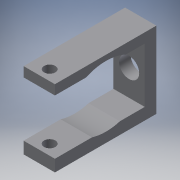
# Autodesk Inventor part: amt_dragster
Saved by Autodesk Inventor 2019 (Build 230136000, 136)
## iProperties
Created: 2024-05-02
Part Number: amt_dragster
Material: Generisch
Document SubType Name: Modeling
Designer: nic
Density: 1 g/cm^3
Appearance: Vorgabe
Author: nic
Autodesk Inventor part; units mm, degrees
ref_plane "YZ Plane" through (0, 0, 0) normal (1, 0, 0) x (0, 1, 0)
ref_plane "XZ Plane" through (0, 0, 0) normal (0, 1, 0) x (-1, 0, 0)
ref_plane "XY Plane" through (0, 0, 0) normal (0, 0, 1) x (1, 0, 0)
sketch "Skizze1" plane through (0, 0, 0) normal (0, 0, 1) x (1, 0, 0)
  line L0 (16.6415, 9.8457) -> (8.5751, 9.8457)
  line L1 (8.5751, 9.8457) -> (8.5751, -9.8457)
  line L2 (8.5751, -9.8457) -> (16.6415, -9.8457)
  line L3 (16.6415, -9.8457) -> (16.6415, 9.8457)
  line L4 (16.6415, 9.8457) -> (8.5751, -9.8457) construction
  line L5 (8.5751, 9.8457) -> (16.6415, -9.8457) construction
  circle A0 centre (12.6083, 0) radius 2.6
  point P0 (0, 0)
  dimension "d0" = 5.2
  constraints: 12 end point, 2 midpoint, 2 parallel, 1 centre point, 1 coincident, 1 horizontal, 1 perpendicular
  measures "d0" diameter of A0
extrude "Extrusion1" add sketch "Skizze1" along normal blind 3
sketch "Skizze2" plane through (0, 0, 3) normal (0, 0, 1) x (1, 0, 0)
  circle A0 centre (12.6083, 0) radius 2.6 construction
  line L0 (16.6415, 9.8457) -> (8.5751, 9.8457) construction
  line L1 (8.5751, 9.8457) -> (8.5751, -9.8457) construction
  line L2 (8.5751, -9.8457) -> (16.6415, -9.8457) construction
  line L3 (16.6415, -9.8457) -> (16.6415, 9.8457) construction
  line L4 (8.5751, 9.8457) -> (8.5751, -9.8457) projected
  line L5 (16.6415, -9.8457) -> (8.5751, -9.8457)
  line L6 (8.5751, -9.8457) -> (8.5751, -6.7929)
  line L7 (8.5751, -6.7929) -> (16.6415, -6.7929)
  line L8 (16.6415, -6.7929) -> (16.6415, -9.8457)
  line L9 (16.6415, -9.8457) -> (16.6415, 9.8457) projected
  line L10 (8.5751, 9.8457) -> (16.6415, 9.8457)
  line L11 (16.6415, 9.8457) -> (16.6415, 7.3365)
  line L12 (16.6415, 7.3365) -> (8.5751, 7.3365)
  line L13 (8.5751, 7.3365) -> (8.5751, 9.8457)
  point P0 (0, 0)
  constraints: 16 end point, 4 parallel, 2 horizontal, 2 perpendicular, 2 point on line
extrude "Extrusion2" add sketch "Skizze2" along normal blind 25 contours L10 L9 L12 L4 | L7 L8 L5 L4
sketch "Skizze3" plane through (8.5751, 7.3365, 3) normal (0, -1, 0) x (1, 0, 0)
  line L0 (8.0665, 0) -> (0, 0) projected
  line L1 (8.0665, 0) -> (8.0665, 25) projected
  line L2 (0, 25) -> (8.0665, 25) projected
  line L3 (0, 0) -> (0, 25) projected
  circle A0 centre (4.0332, 20.469) radius 1.4552
  point P0 (-8.5751, -3)
  constraints: 1 centre point
extrude "Extrusion3" cut sketch "Skizze3" along normal through all both and the other way through all contours A0
sketch "Skizze4" plane through (8.5751, -9.8457, 0) normal (0, -1, 0) x (1, 0, 0)
  line L0 (8.0665, 3) -> (8.0665, 28) projected
  line L1 (0, 3) -> (0, 28) projected
  line L2 (8.0665, 28) -> (0, 28)
  line L3 (0, 28) -> (0, 26.1511)
  line L4 (0, 26.1511) -> (8.0665, 26.1511)
  line L5 (8.0665, 26.1511) -> (8.0665, 28)
  point P0 (-8.5751, 0)
  constraints: 8 end point, 2 parallel, 1 horizontal, 1 perpendicular, 1 point on line
extrude "Extrusion4" cut sketch "Skizze4" against normal through all
sketch "Skizze5" plane through (16.6415, -9.8457, 0) normal (1, 0, 0) x (0, 0, -1)
  ellipse E0 centre (-12.9855, 10.4116) end of major axis (-22.9331, 10.4116) minor radius 7.8919
  point P0 (0, 9.8457)
  constraints: 2 other
extrude "Extrusion5" cut sketch "Skizze5" along normal through all both and the other way through all
